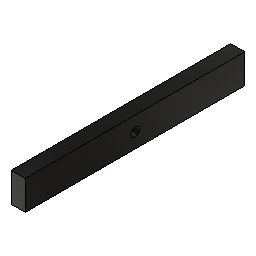
CameraLevelLock v2 (Autodesk Fusion 360 design; units mm, degrees)
Autodesk Fusion 360 part; units mm, degrees
sketch "Sketch1" plane through (0, 0, 0) normal (1, 0, 0) x (0, 1, 0)
  line L0 (-37.3, 5) -> (37.3, 5)
  line L1 (37.3, 5) -> (37.3, -5)
  line L2 (37.3, -5) -> (-37.3, -5)
  line L3 (-37.3, -5) -> (-37.3, 5)
  line L4 (0, 0) -> (0, 5) construction
  line L5 (0, 0) -> (-37.3, 0) construction
  circle A0 centre (0, 0) radius 1.5
  point P0 (0, 5)
  point P1 (-37.3, 0)
  dimension "d1" = 3
  dimension "d2" = 10
  dimension "d3" = 74.6
  constraint horizontal L0
  constraint vertical L1
  constraint horizontal L2
  constraint vertical L3
  constraint midpoint L0 P0
  constraint midpoint L3 P1
  constraint coincident L4.start L5.start
  constraint coincident P0 L4.end
  constraint coincident P1 L5.end
  constraint horizontal L5
  constraint vertical L4
  measures "d1" diameter of A0
  measures "d2" distance of L0.start L2.end
  measures "d3" distance of L0.start L0.end
extrude "Extrude1" add sketch "Sketch1" along normal blind 4.8
